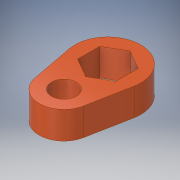
# Autodesk Inventor part: Piston Nut trap
Saved by Autodesk Inventor 2018.1 (Build 221171000, 171)
## iProperties
Created: 2013-10-18
Part Number: Piston Nut trap
Material: ABS Plastic
Document SubType Name: Modeling
Designer: Gabriel Smolnycki
Mass: 0.612143 g
Surface Area: 6.69271 cm^2
Volume: 0.577493 cm^3
Density: 1.06 g/cm^3
Appearance: Smooth - Light Orange
Author: Gabriel Smolnycki
Sending System: SolidWorks 2017
Last Author: Gabriel Smolnycki
Last Saved: 2017-09-14
Autodesk Inventor part; units mm, degrees
ref_plane "YZ Plane" through (0, 0, 0) normal (1, 0, 0) x (0, 1, 0)
ref_plane "XZ Plane" through (0, 0, 0) normal (0, 1, 0) x (-1, 0, 0)
ref_plane "XY Plane" through (0, 0, 0) normal (0, 0, 1) x (1, 0, 0)
sketch "Sketch1" plane through (0, 0, 0) normal (0, 1, 0) x (-1, 0, 0)
  line L0 (3.5, 2.0207) -> (0, 4.0415)
  line L1 (0, 4.0415) -> (-3.5, 2.0207)
  line L2 (-3.5, 2.0207) -> (-3.5, -2.0207)
  line L3 (-3.5, -2.0207) -> (0, -4.0415)
  line L4 (-4.4202, 8.8438) -> (-5.8936, 1.125)
  arc A0 (4.4202, 8.8438) -> (-4.4202, 8.8438) centre (0, 8) ccw
  line L5 (5.8936, 1.125) -> (4.4202, 8.8438)
  line L6 (0, -4.0415) -> (3.5, -2.0207)
  arc A1 (-5.8936, 1.125) -> (5.8936, 1.125) centre (0, 0) ccw
  line L7 (3.5, -2.0207) -> (3.5, 2.0207)
  constraints: 16 end point, 6 equal length, 4 point on circle, 2 centre point, 2 vertical
extrude "Extrusion1" add sketch "Sketch1" along normal blind 5
sketch "Sketch2" plane through (0, 5, 0) normal (0, 1, 0) x (1, 0, 0)
  point P0 (0, -8)
hole "Hole1" at (0, 5, 8) direction (0, -1, 0) diameter 4.5 depth 5 tip angle 118
body "Solid3"
